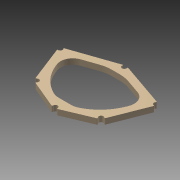
# Autodesk Inventor part: section1
Saved by Autodesk Inventor 2015 (Build 190159000, 159)
## iProperties
Created: 2017-09-23
Part Number: section1
Material: Polyethylene, High Density
Document SubType Name: Modeling
Designer: Mimoja
Density: 0.952 g/cm^3
Appearance: Smooth - Off-White
Mass: 294.208 g
Surface Area: 626.554 cm^2
Volume: 309.042 cm^3
Author: Mimoja
Autodesk Inventor part; units mm, degrees
ref_plane "YZ Plane" through (0, 0, 0) normal (1, 0, 0) x (0, 1, 0)
ref_plane "XZ Plane" through (0, 0, 0) normal (0, 1, 0) x (-1, 0, 0)
ref_plane "XY Plane" through (0, 0, 0) normal (0, 0, 1) x (1, 0, 0)
sketch "Sketch1" plane through (0, 0, 0) normal (0, 0, 1) x (1, 0, 0)
  line L0 (0, 27.432) -> (-109.1184, 73.152)
  line L1 (-109.1184, 73.152) -> (-161.8488, 208.4832)
  line L2 (-161.8488, 208.4832) -> (0, 264.2616)
  line L3 (0, 562.8605) -> (0, -145.2705) construction
  line L4 (0, 264.2616) -> (0, 27.432)
  point P0 (0, 0)
  dimension "d9" = 264.2616
  dimension "d11" = 161.8488
  dimension "d15" = 208.4832
  dimension "d20" = 109.1184
  dimension "d22" = 73.152
  dimension "d39" = 0
  dimension "d41" = 0
  dimension "d42" = 27.432
  constraints: 10 end point, 1 vertical
  measures "d9" distance of point (0, 0) L2.end
  measures "d11" horizontal distance of point (0, 0) L1.end
  measures "d15" vertical distance of point (0, 0) L1.end
  measures "d20" horizontal distance of point (0, 0) L0.end
  measures "d22" vertical distance of point (0, 0) L0.end
  measures "d39" horizontal distance of point (0, 0) L2.end
  measures "d41" horizontal distance of point (0, 0) L0.start
  measures "d42" distance of point (0, 0) L0.start
extrude "Extrusion4" add sketch "Sketch1" along normal blind 18
hole "Hole2" at (0.0182, 257.4006, 18) direction (0, 0, -1) diameter 15 end through all
hole "Hole3" at (-155.3023, 205.1164, 18) direction (0, 0, -1) diameter 15 end through all
hole "Hole4" at (-104.3588, 77.9489, 18) direction (0, 0, -1) diameter 15 end through all
hole "Hole5" at (0.2097, 34.0914, 18) direction (0, 0, -1) diameter 15 end through all
fillet "Fillet7" radius 1.5 1 edges at (-5.647, 262.3155, 9)
fillet "Fillet8" radius 1 1 edges at (-152.0327, 211.8661, 9)
fillet "Fillet9" radius 1 1 edges at (-157.7785, 198.0369, 9)
fillet "Fillet10" radius 2 1 edges at (-111.6584, 79.6709, 9)
fillet "Fillet11" radius 2 1 edges at (-102.9745, 70.5777, 9)
fillet "Fillet12" radius 2 1 edges at (-6.056, 29.9694, 9)
sketch "Sketch5" plane through (0, 0, 18) normal (0, 0, 1) x (1, 0, 0)
  line L0 (0, 41.5885) -> (0, 249.9006) projected
  line L1 (-91.2304, 90.5943) -> (-131.73, 194.5356)
  line L2 (-131.73, 194.5356) -> (-30, 229.5951)
  line L3 (-30, 229.5951) -> (0, 229.5951)
  line L4 (-9.1769, 261.0989) -> (-150.1114, 212.5283) projected
  line L5 (-157.1008, 196.2976) -> (-113.2116, 83.657) projected
  line L6 (-98.9493, 68.8912) -> (-10.0438, 31.6403) projected
  line L7 (-91.2304, 90.5943) -> (-30, 64.9391)
  line L8 (-30, 64.9391) -> (0, 64.9391)
  point P0 (0, 0)
  dimension "d148" = 23
  dimension "d149" = 23
  dimension "d151" = 23
  dimension "d152" = 30
  dimension "d153" = 30
  constraints: 10 end point, 3 parallel, 2 point on line, 1 horizontal, 1 perpendicular
  measures "d148" distance between parallel lines of L2 L4
  measures "d149" distance between parallel lines of L1 L5
  measures "d151" distance between parallel lines of L6 L7
  measures "d152" distance from line of L0 L7.end
  measures "d153" distance from line of L0 L2.end
extrude "Extrusion5" cut sketch "Sketch5" against normal through all
fillet "Fillet14" radius 40 1 edges at (-131.73, 194.5356, 9)
fillet "Fillet15" radius 100 1 edges at (-30, 229.5951, 9)
fillet "Fillet16" radius 150 1 edges at (-91.2304, 90.5943, 9)
fillet "Fillet17" radius 50 1 edges at (-30, 64.9391, 9)
mirror "Mirror2" about plane through (0, 0, 0) normal (1, 0, 0)
body "Solid4"
